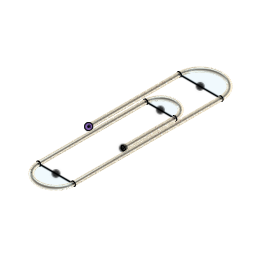
PaperClip (Autodesk Fusion 360 design; units mm, degrees)
part number: 2025-07-13-15-04-41-414
Autodesk Fusion 360 part; units mm, degrees
sketch "Paper clip path" plane through (0, 0, 0) normal (0, 0, 1) x (1, 0, 0)
  line L0 (0, 0) -> (0, 16.25)
  line L1 (0, 16.25) -> (7.5, 16.25)
  line L2 (7.5, 16.25) -> (7.5, -10.25)
  line L3 (7.5, -10.25) -> (1.25, -10.25)
  line L4 (1.25, -10.25) -> (1.25, 9)
  line L5 (1.25, 9) -> (6.45, 9)
  line L6 (6.45, 9) -> (6.45, -0.25)
  arc A0 (7.5, 16.25) -> (0, 16.25) centre (3.75, 16.25) ccw
  arc A1 (6.45, 9) -> (1.25, 9) centre (3.85, 9) ccw
  arc A2 (1.25, -10.25) -> (7.5, -10.25) centre (4.375, -10.25) ccw
  dimension "d1" = 16.25
  dimension "d2" = 7.5
  dimension "d3" = 26.5
  dimension "d4" = 6.25
  dimension "d5" = 19.25
  dimension "d6" = 5.2
  dimension "d7" = 9.25
  constraint coincident L0.start origin
  constraint vertical L0
  constraint perpendicular L0 L1
  constraint perpendicular L1 L2
  constraint perpendicular L2 L3
  constraint perpendicular L3 L4
  constraint perpendicular L4 L5
  constraint perpendicular L5 L6
  constraint tangent L0 A0
  constraint tangent L4 A1
  constraint tangent L4 A2
  measures "d1" distance of L0.start L0.end
  measures "d2" distance of L0.end L1.end
  measures "d3" distance of L1.end L2.end
  measures "d4" distance of L2.end L3.end
  measures "d5" distance of L3.end L4.end
  measures "d6" distance of L4.end L5.end
  measures "d7" distance of L5.end L6.end
sketch "hole" plane through (0, 0, 0) normal (0, 1, 0) x (1, 0, 0)
  circle A0 centre (0, 0) radius 0.375
  dimension "d8" = 0.75
  constraint coincident A0.centre origin
  measures "d8" diameter of A0
sweep "Sweep1" add profiles "hole" path "Paper clip path" along L0 A0 L2 A2 L4 A1 L6 section 1
